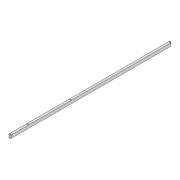
# Autodesk Inventor part: Part_13
Saved by Autodesk Inventor 2022 (Build 260153000, 153)
## iProperties
Created: 2022-05-03
Part Number: Part_13
Material: Generic
Document SubType Name: Modeling
Designer: dell
Density: 1 g/cm^3
Appearance: Default
Author: dell
Autodesk Inventor part; units mm, degrees
ref_plane "YZ Plane" through (0, 0, 0) normal (1, 0, 0) x (0, 1, 0)
ref_plane "XZ Plane" through (0, 0, 0) normal (0, 1, 0) x (-1, 0, 0)
ref_plane "XY Plane" through (0, 0, 0) normal (0, 0, 1) x (1, 0, 0)
sketch "Sketch1" plane through (0, 0, 0) normal (0, 1, 0) x (-1, 0, 0)
  line L0 (0, 0) -> (0, -435.595) construction
  line L1 (-3, 0) -> (-3, -435.595)
  line L2 (3, -435.595) -> (3, 0)
  arc A0 (3, 0) -> (-3, 0) centre (0, 0) ccw
  arc A1 (-3, -435.595) -> (3, -435.595) centre (0, -435.595) ccw
  circle A2 centre (0, 0) radius 1.5
  circle A3 centre (0, -435.595) radius 1.5
  circle A4 centre (0, -47.52) radius 1.5
  circle A5 centre (0, -164.378) radius 1.5
  point P0 (0, -217.7975)
  dimension "d0" = 6
  dimension "d1" = 435.595
  dimension "d2" = 3
  dimension "d3" = 3
  dimension "d20" = 3
  dimension "d21" = 47.52
  dimension "d22" = 3
  dimension "d23" = 164.378
  constraints: 8 end point, 6 centre point, 4 point on circle, 4 tangent, 2 coincident, 2 point on line, 1 midpoint, 1 parallel, 1 vertical
  measures "d0" diameter of A1
  measures "d1" distance of L0.end L0.start
  measures "d2" diameter of A2
  measures "d3" diameter of A3
  measures "d20" diameter of A4
  measures "d21" distance of L0.start A4.centre
  measures "d22" diameter of A5
  measures "d23" distance of L0.start A5.centre
extrude "Extrusion1" add sketch "Sketch1" along normal blind 8
body "Solid1"
